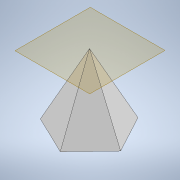
# Autodesk Inventor part: largePart
Saved by Autodesk Inventor 2021 (Build 250183000, 183)
## iProperties
Created: 2020-11-29
Part Number: largePart
Material: Generic
Document SubType Name: Modeling
Designer: awitc
Density: 1 g/cm^3
Appearance: Default
Author: awitc
Autodesk Inventor part; units mm, degrees
ref_plane "YZ Plane" through (0, 0, 0) normal (1, 0, 0) x (0, 1, 0)
ref_plane "XY Plane" through (0, 0, 0) normal (0, 0, 1) x (1, 0, 0)
sketch "Sketch1" plane through (0, 0, 0) normal (0, 1, 0) x (-1, 0, 0)
  line L0 (30.7278, -29.4078) -> (-18.4731, -38.3114)
  line L1 (-18.4731, -38.3114) -> (-42.1448, 5.7301)
  line L2 (-42.1448, 5.7301) -> (-7.5738, 41.8528)
  line L3 (-7.5738, 41.8528) -> (37.4639, 20.1364)
  line L4 (37.4639, 20.1364) -> (30.7278, -29.4078)
  point P0 (0, 0)
  point P1 (0, 0)
  constraints: 10 end point, 11 other
ref_plane "Work Plane1" through (0, 80, 0) normal (0, 1, 0) x (-1, 0, 0)
sketch "Sketch2" plane through (0, 80, 0) normal (0, 1, 0) x (-1, 0, 0)
  point P0 (0, 0)
  point P1 (0, 0)
  constraints: 1 coincident
loft "Loft1" add profiles "Sketch1" section 2 point at (0, 80, 0)
body "Solid1"
